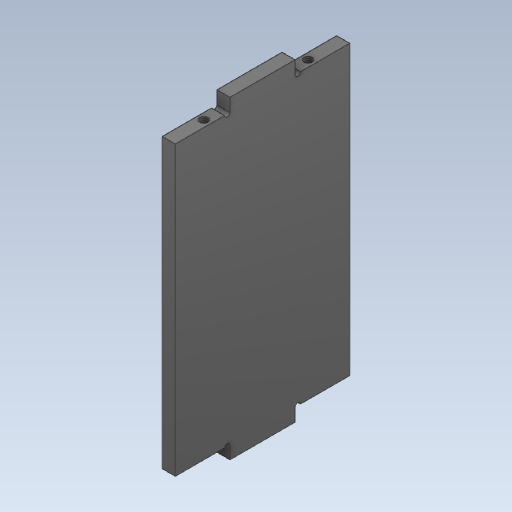
# Autodesk Inventor part: Cockpit_front_frame
Saved by Autodesk Inventor 2020.4 (Build 244396000, 396)
## iProperties
Created: 2022-01-04
Part Number: Cockpit_front_frame
Material: アセタール樹脂、黒
Document SubType Name: Modeling
Designer: Masato Kubotera
Density: 1.425 g/cm^3
Appearance: 滑らか - 黒
Mass: 54.5952 g
Surface Area: 173.687 cm^2
Volume: 38.3125 cm^3
Author: Masato Kubotera
Autodesk Inventor part; units mm, degrees
ref_plane "XZ Plane" through (0, 0, 0) normal (0, 1, 0) x (-1, 0, 0)
ref_plane "XY Plane" through (0, 0, 0) normal (0, 0, 1) x (1, 0, 0)
derived "Cockpit_side_frame.ipt"
sketch "スケッチ1" plane through (0, 0, 0) normal (0, 1, 0) x (-1, 0, 0)
  line L0 (-60, 36) -> (60, 36) construction
  line L1 (60, 36) -> (60, -36) construction
  line L2 (60, -36) -> (-60, -36) construction
  line L3 (-60, -36) -> (-60, 36) construction
  line L4 (-60, 36) -> (60, -36) construction
  line L5 (60, 36) -> (-60, -36) construction
  line L6 (-52.5, 6) -> (52.5, 6) construction
  line L7 (52.5, 6) -> (52.5, 1) construction
  line L8 (52.5, 1) -> (-52.5, 1) construction
  line L9 (-52.5, 1) -> (-52.5, 6) construction
  line L10 (-52.5, 6) -> (52.5, 1) construction
  line L11 (52.5, 6) -> (-52.5, 1) construction
  line L12 (0, 36) -> (0, -36) construction
  line L13 (-57.5, 33.5) -> (-52.5, 33.5) construction
  line L14 (-52.5, 33.5) -> (-52.5, -33.5) construction
  line L15 (-52.5, -33.5) -> (-57.5, -33.5) construction
  line L16 (-57.5, -33.5) -> (-57.5, 33.5) construction
  line L17 (-57.5, 33.5) -> (-52.5, -33.5) construction
  line L18 (-52.5, 33.5) -> (-57.5, -33.5) construction
  line L19 (-55, 36) -> (-60, 31)
  line L20 (-60, 0) -> (60, 0) construction
  line L21 (-46.5, 41) -> (32.5, 41) construction
  line L22 (32.5, 41) -> (32.5, 11) construction
  line L23 (32.5, 11) -> (-46.5, 11) construction
  line L24 (-46.5, 11) -> (-46.5, 41) construction
  line L25 (-46.5, 41) -> (32.5, 11) construction
  line L26 (32.5, 41) -> (-46.5, 11) construction
  line L27 (-55, -36) -> (-60, -31)
  line L28 (-60, 31) -> (-60, -31)
  line L29 (55, -36) -> (60, -31)
  line L30 (-52.5, -28.5) -> (52.5, -28.5) construction
  line L31 (52.5, -28.5) -> (52.5, -33.5) construction
  line L32 (52.5, -33.5) -> (-52.5, -33.5) construction
  line L33 (-52.5, -33.5) -> (-52.5, -28.5) construction
  line L34 (-52.5, -28.5) -> (52.5, -33.5) construction
  line L35 (52.5, -28.5) -> (-52.5, -33.5) construction
  line L36 (-25, -28.5) -> (-25, -33.5) construction
  line L37 (-55, -33.5) -> (-55, 33.5) construction
  line L38 (-57.5, 12.5) -> (-52.5, 12.5) construction
  line L39 (-57.55, 12.55) -> (-52.45, 12.55)
  line L40 (-52.45, 12.55) -> (-52.45, -12.55)
  line L41 (-52.45, -12.55) -> (-57.55, -12.55)
  line L42 (-57.55, -12.55) -> (-57.55, 12.55)
  line L43 (-57.55, 12.55) -> (-52.45, -12.55) construction
  line L44 (-52.45, 12.55) -> (-57.55, -12.55) construction
  arc A0 (-52.45, 11.0651) -> (-53.9349, 12.55) centre (-53.1925, 11.8075) ccw
  circle A1 centre (-55, 20) radius 1.6
  circle A2 centre (-55, -20) radius 1.6
  arc A3 (-53.9349, -12.55) -> (-52.45, -11.0651) centre (-53.1925, -11.8075) ccw
  line L45 (-57.5, -12.5) -> (-52.5, -12.5) construction
  arc A4 (-56.0651, 12.55) -> (-57.55, 11.0651) centre (-56.8075, 11.8075) ccw
  arc A5 (-57.55, -11.0651) -> (-56.0651, -12.55) centre (-56.8075, -11.8075) ccw
  line L46 (-52.5, -31) -> (52.5, -31) construction
  line L47 (-25.05, -33.5) -> (-25.05, -28.45)
  line L48 (-25.05, -28.45) -> (25.05, -28.45)
  circle A6 centre (-32.5, -31) radius 1.6
  circle A7 centre (32.5, -31) radius 1.6
  line L49 (25, -28.5) -> (25, -33.5) construction
  line L50 (52.5, 33.5) -> (57.5, 33.5) construction
  line L51 (57.5, 33.5) -> (57.5, -33.5) construction
  line L52 (57.5, -33.5) -> (52.5, -33.5) construction
  line L53 (52.5, -33.5) -> (52.5, 33.5) construction
  line L54 (52.5, 33.5) -> (57.5, -33.5) construction
  line L55 (57.5, 33.5) -> (52.5, -33.5) construction
  line L56 (52.5, 0) -> (57.5, 0) construction
  line L57 (52.5, -12.5) -> (57.5, -12.5) construction
  line L58 (55, -33.5) -> (55, 33.5) construction
  circle A8 centre (55, -20) radius 1.6
  line L59 (60, -12.55) -> (52.45, -12.55)
  line L60 (52.45, -12.55) -> (52.45, 12.55)
  arc A9 (52.45, -11.0651) -> (53.9349, -12.55) centre (53.1925, -11.8075) ccw
  line L61 (60, 12.55) -> (52.45, 12.55)
  arc A10 (53.9349, 12.55) -> (52.45, 11.0651) centre (53.1925, 11.8075) ccw
  line L62 (52.5, 12.5) -> (57.5, 12.5) construction
  circle A11 centre (55, 20) radius 1.6
  arc A12 (-23.5651, -28.45) -> (-25.05, -29.9349) centre (-24.3075, -29.1925) ccw
  arc A13 (25.05, -29.9349) -> (23.5651, -28.45) centre (24.3075, -29.1925) ccw
  circle A14 centre (-55, 20) radius 3
  circle A15 centre (-32.5, -31) radius 3
  circle A16 centre (-55, -20) radius 3
  circle A17 centre (32.5, -31) radius 3
  line L63 (-25.05, -33.5) -> (-27.55, -36)
  line L64 (-55, -36) -> (-27.55, -36)
  line L65 (25.05, -33.5) -> (27.55, -36)
  line L66 (25.05, -33.5) -> (25.05, -28.45)
  line L67 (55, -36) -> (27.55, -36)
  line L68 (25.05, 6.05) -> (-25.05, 6.05)
  line L69 (-25.05, 6.05) -> (-25.05, 0.95)
  line L70 (-25.05, 0.95) -> (25.05, 0.95)
  line L71 (25.05, 0.95) -> (25.05, 6.05)
  line L72 (25.05, 6.05) -> (-25.05, 0.95) construction
  line L73 (-25.05, 6.05) -> (25.05, 0.95) construction
  line L74 (-25, 6) -> (-25, 1) construction
  arc A18 (-23.5651, 6.05) -> (-25.05, 4.5651) centre (-24.3075, 5.3075) ccw
  line L75 (52.5, 3.5) -> (-52.5, 3.5) construction
  circle A19 centre (-32.5, 3.5) radius 1.6
  line L76 (25, 6) -> (25, 1) construction
  arc A20 (25.05, 4.5651) -> (23.5651, 6.05) centre (24.3075, 5.3075) ccw
  circle A21 centre (32.5, 3.5) radius 1.6
  arc A22 (-25.05, 2.4349) -> (-23.5651, 0.95) centre (-24.3075, 1.6925) ccw
  arc A23 (23.5651, 0.95) -> (25.05, 2.4349) centre (24.3075, 1.6925) ccw
  line L77 (60, 31) -> (60, 12.55)
  line L78 (60, -12.55) -> (60, -31)
  circle A24 centre (-32.5, 3.5) radius 3
  circle A25 centre (55, -20) radius 3
  circle A26 centre (55, 20) radius 3
  circle A27 centre (32.5, 3.5) radius 3
  line L79 (60, 31) -> (60, 41)
  line L80 (18, 36) -> (-55, 36)
  line L81 (60, 41) -> (55, 46)
  line L82 (55, 46) -> (50, 46)
  line L83 (50, 46) -> (50, 41)
  line L84 (50, 41) -> (39, 41)
  line L85 (39, 41) -> (39, 46)
  line L86 (39, 46) -> (29, 46)
  line L87 (29, 46) -> (29, 41)
  line L88 (29, 41) -> (18, 41)
  line L89 (18, 41) -> (18, 36)
  circle A28 centre (-45, 0) radius 1.75
  line L90 (34, 46) -> (34, 41) construction
  point P0 (0, 0)
  point P1 (0, 3.5)
  point P2 (-55, 0)
  point P3 (-55, 0)
  point P4 (-7, 26)
  point P5 (0, -31)
  point P6 (0, 3.5)
  point P7 (51.9559, 36)
  dimension "d1" = 67
  dimension "d2" = 25
  dimension "d3" = 40
  dimension "d20" = 52.5
  dimension "d21" = 5
  measures "d1" distance of L15.end L13.start
  measures "d2" distance of L45.start L38.start
  measures "d3" distance of A16.centre A1.centre
  measures "d20" horizontal distance of L32.end L12.end
  measures "d21" distance of L14.end L15.end
ref_plane "作業平面1" through (52.5, 0, 0) normal (1, 0, 0) x (0, 1, 0)
sketch "スケッチ3" plane through (52.5, 0, 0) normal (1, 0, 0) x (0, 1, 0)
  line L0 (-110.5, 33.5) -> (0, 33.5)
  line L1 (0, -33.5) -> (-110.5, -33.5)
  line L2 (-110.5, 33.5) -> (0, -33.5) construction
  line L3 (0, 33.5) -> (-110.5, -33.5) construction
  line L4 (-116.0272, 0) -> (0, 0) construction
  line L5 (-55.25, 33.5) -> (-55.25, -33.5) construction
  line L6 (0, 12.5) -> (5, 12.5)
  line L7 (5, 12.5) -> (5, -12.5)
  line L8 (0, -12.5) -> (5, -12.5)
  arc A0 (0, 14.6) -> (0, 12.5) centre (0, 13.55) ccw
  line L9 (0, 33.5) -> (0, 14.6)
  line L10 (0, -14.6) -> (0, -33.5)
  arc A1 (0, -12.5) -> (0, -14.6) centre (0, -13.55) ccw
  line L11 (-110.5, 33.5) -> (-110.5, 14.6)
  arc A2 (-110.5, 12.5) -> (-110.5, 14.6) centre (-110.5, 13.55) ccw
  line L12 (-110.5, 12.5) -> (-115.5, 12.5)
  line L13 (-115.5, 12.5) -> (-115.5, -12.5)
  line L14 (-110.5, -12.5) -> (-115.5, -12.5)
  arc A3 (-110.5, -14.6) -> (-110.5, -12.5) centre (-110.5, -13.55) ccw
  line L15 (-110.5, -14.6) -> (-110.5, -33.5)
  point P0 (-55.25, 0)
  point P1 (0, 12.55)
  point P2 (0, 12.55)
  point P3 (0, 12.55)
  point P4 (0, -12.5)
  point P5 (0, -12.5)
  point P6 (0, -12.5)
  point P7 (-55.25, 0)
  dimension "d12" = 67
  dimension "d13" = 110.5
  dimension "d14" = 25
  dimension "d15" = 5
  dimension "d16" = 1.05
  constraints: 32 end point, 13 symmetric about line, 8 point on circle, 8 point on line, 5 midpoint, 4 centre point, 2 horizontal, 2 perpendicular, 1 coincident, 1 collinear, 1 parallel, 1 tangent, 1 vertical, 3 other
  measures "d12" distance of L3.end L0.start
  measures "d13" distance of L0.start L9.start
  measures "d14" distance of L7.start L7.end
  measures "d15" distance of L6.start L7.start
  measures "d16" radius of A0
extrude "押し出し2" add sketch "スケッチ3" along normal blind 5
hole "穴1" at (55, 0, 20) at (55, 0, -20) direction (0, -1, 0) diameter 3.242 depth 5 tip angle 118 thread size "M4x0.7" class "6H" standard "ISO Metric profile"
equation "\"d12\" = d17"
equation "\"d14\" = d2"
equation "\"d22\" = d21"
equation "\"d11\" = d19"
equation "\"d19\" = d20"
equation "\"d17\" = 67"
